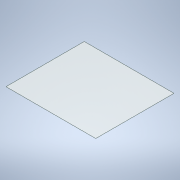
# Autodesk Inventor part: glass
Saved by Autodesk Inventor 2021 (Build 250183000, 183)
## iProperties
Created: 2021-04-11
Part Number: glass
Material: Glass
Document SubType Name: Modeling
Designer: victo
Density: 2.18 g/cm^3
Appearance: Clear
Author: victo
Autodesk Inventor part; units mm, degrees
ref_plane "YZ Plane" through (0, 0, 0) normal (1, 0, 0) x (0, 1, 0)
ref_plane "XZ Plane" through (0, 0, 0) normal (0, 1, 0) x (-1, 0, 0)
ref_plane "XY Plane" through (0, 0, 0) normal (0, 0, 1) x (1, 0, 0)
sketch "Sketch1" plane through (0, 0, 0) normal (0, 1, 0) x (-1, 0, 0)
  line L0 (0, 0) -> (555, 0)
  line L1 (555, 0) -> (555, -484)
  line L2 (555, -484) -> (0, -484)
  line L3 (0, -484) -> (0, 0)
  dimension "d0" = 484
  dimension "d1" = 555
  constraints: 8 end point, 2 parallel, 1 horizontal, 1 perpendicular
  measures "d0" distance of L0.end L1.end
  measures "d1" distance of L1.end L2.end
extrude "Extrusion1" add sketch "Sketch1" along normal blind 1
body "Solid1"
